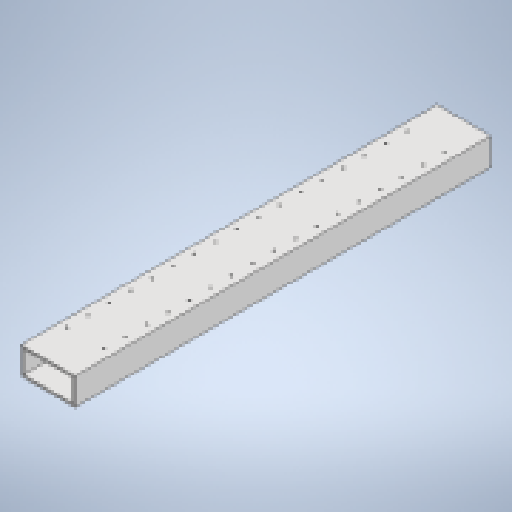
# Autodesk Inventor part: HORIZONTALTUBE
Saved by Autodesk Inventor 2023 (Build 270158000, 158)
## iProperties
Created: 2022-05-02
Part Number: HORIZONTALTUBE
Material: Generic
Document SubType Name: Modeling
Designer: plebbb
Density: 1 g/cm^3
Appearance: Default
Author: plebbb
Autodesk Inventor part; units mm, degrees
ref_plane "YZ Plane" through (0, 0, 0) normal (1, 0, 0) x (0, 1, 0)
ref_plane "XZ Plane" through (0, 0, 0) normal (0, 1, 0) x (-1, 0, 0)
ref_plane "XY Plane" through (0, 0, 0) normal (0, 0, 1) x (1, 0, 0)
sketch "Sketch1" plane through (0, 0, 0) normal (0, 0, 1) x (1, 0, 0)
  line L0 (0, 0) -> (152.4, 0)
  line L1 (152.4, 0) -> (152.4, 76.2)
  line L2 (152.4, 76.2) -> (0, 76.2)
  line L3 (0, 76.2) -> (0, 0)
  dimension "d0" = 152.4
  dimension "d1" = 76.2
  constraints: 8 end point, 2 parallel, 1 horizontal, 1 perpendicular
  measures "d0" distance of L1.end L2.end
  measures "d1" distance of L0.end L1.end
extrude "Extrusion1" add sketch "Sketch1" along normal blind 1174.2928
shell "Shell1" thickness 6.35 removed faces 2 at (50.8, 50.8, 0) at (50.8, 50.8, 1174.2928)
sketch "Sketch2" plane through (0, 76.2, 0) normal (0, 1, 0) x (1, 0, 0)
  circle A0 centre (124.9, -1067.1428) radius 3 projected
  circle A1 centre (124.9, -1007.1428) radius 3 projected
  circle A2 centre (124.9, -947.1428) radius 3 projected
  circle A3 centre (124.9, -887.1428) radius 3 projected
  circle A4 centre (124.9, -827.1428) radius 3 projected
  circle A5 centre (124.9, -767.1428) radius 3 projected
  circle A6 centre (124.9, -707.1428) radius 3 projected
  circle A7 centre (124.9, -647.1428) radius 3 projected
  circle A8 centre (124.9, -587.1428) radius 3 projected
  circle A9 centre (124.9, -527.1428) radius 3 projected
  circle A10 centre (124.9, -467.1428) radius 3 projected
  circle A11 centre (124.9, -407.1428) radius 3 projected
  circle A12 centre (124.9, -347.1428) radius 3 projected
  circle A13 centre (124.9, -287.1428) radius 3 projected
  circle A14 centre (124.9, -227.1428) radius 3 projected
  circle A15 centre (124.9, -167.1428) radius 3 projected
  circle A16 centre (124.9, -107.1428) radius 3 projected
  line L0 (114.9, -87.1428) -> (134.9, -87.1428) projected
  line L1 (134.9, -87.1428) -> (134.9, -1087.1428) projected
  line L2 (114.9, -1087.1428) -> (134.9, -1087.1428) projected
  line L3 (114.9, -87.1428) -> (114.9, -1087.1428) projected
  circle A17 centre (19.9, -1067.1428) radius 3 projected
  circle A18 centre (19.9, -1007.1428) radius 3 projected
  circle A19 centre (19.9, -947.1428) radius 3 projected
  circle A20 centre (19.9, -887.1428) radius 3 projected
  circle A21 centre (19.9, -827.1428) radius 3 projected
  circle A22 centre (19.9, -767.1428) radius 3 projected
  circle A23 centre (19.9, -707.1428) radius 3 projected
  circle A24 centre (19.9, -647.1428) radius 3 projected
  circle A25 centre (19.9, -587.1428) radius 3 projected
  circle A26 centre (19.9, -527.1428) radius 3 projected
  circle A27 centre (19.9, -467.1428) radius 3 projected
  circle A28 centre (19.9, -407.1428) radius 3 projected
  circle A29 centre (19.9, -347.1428) radius 3 projected
  circle A30 centre (19.9, -287.1428) radius 3 projected
  circle A31 centre (19.9, -227.1428) radius 3 projected
  circle A32 centre (19.9, -167.1428) radius 3 projected
  circle A33 centre (19.9, -107.1428) radius 3 projected
  line L4 (9.9, -87.1428) -> (29.9, -87.1428) projected
  line L5 (29.9, -87.1428) -> (29.9, -1087.1428) projected
  line L6 (9.9, -1087.1428) -> (29.9, -1087.1428) projected
  line L7 (9.9, -87.1428) -> (9.9, -1087.1428) projected
  point P0 (0, 0)
extrude "Extrusion2" cut sketch "Sketch2" against normal up to surface (6.35 mm away) contours A0 | A1 | A2 | A3 | A4 | A5 | A6 | A7 | A8 | A9 | A10 | A11 | A12 | A13 | A14 | A15 | A16 | A17 | A18 | A19 | A20 | A21 | A22 | A23 | A24 | A25 | A26 | A27 | A28 | A29 | A30 | A31 | A32 | A33
body "Solid1"
